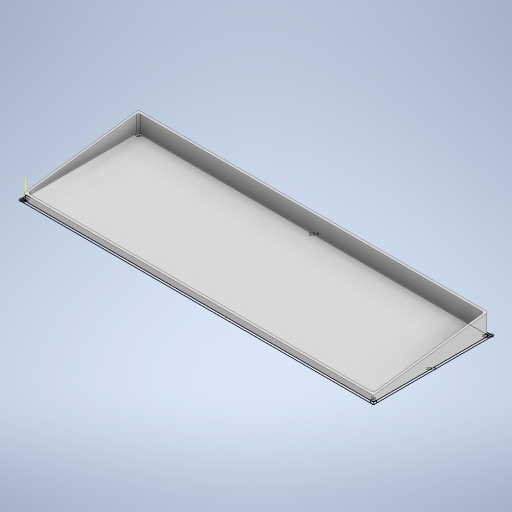
# Autodesk Inventor part: case_in_one
Saved by Autodesk Inventor 2024 (Build 280153000, 153)
## iProperties
Created: 2023-08-03
Part Number: case_in_one
Material: Generic
Document SubType Name: Modeling
Designer: Mika
Density: 1 g/cm^3
Appearance: Default
Author: Mika
Autodesk Inventor part; units mm, degrees
ref_plane "YZ Plane" through (0, 0, 0) normal (1, 0, 0) x (0, 1, 0)
ref_plane "XZ Plane" through (0, 0, 0) normal (0, 1, 0) x (-1, 0, 0)
ref_plane "XY Plane" through (0, 0, 0) normal (0, 0, 1) x (1, 0, 0)
sketch "Sketch1" plane through (0, 0, 0) normal (0, 1, 0) x (-1, 0, 0)
  line L0 (0, 0) -> (-2, 0)
  line L1 (-2, 0) -> (-2, -2)
  line L2 (-2, -2) -> (0, -2)
  line L3 (0, -2) -> (0, 0)
  line L4 (-2, -2) -> (-310.9, -2)
  line L5 (-310.9, -2) -> (-310.9, -103.5)
  line L6 (-308.9, -103.5) -> (-2, -103.5)
  line L7 (-2, -103.5) -> (-2, -2)
  line L8 (-310.9, -103.5) -> (-312.9, -103.5)
  line L9 (-312.9, -103.5) -> (-312.9, -105.5)
  line L10 (-312.9, -105.5) -> (-310.9, -105.5)
  line L11 (-310.9, -105.5) -> (-310.9, -103.5)
  line L12 (-312.9, -105.5) -> (0, -105.5)
  line L13 (0, -105.5) -> (0, 0)
  line L14 (0, 0) -> (-312.9, 0)
  line L15 (-312.9, 0) -> (-312.9, -105.5)
  line L16 (-2, -2) -> (-4, -2)
  line L17 (-4, -2) -> (-4, -4)
  line L18 (-4, -4) -> (-2, -4)
  line L19 (-2, -4) -> (-2, -2)
  line L20 (-2, -103.5) -> (-4, -103.5)
  line L21 (-4, -103.5) -> (-4, -101.5)
  line L22 (-4, -101.5) -> (-2, -101.5)
  line L23 (-2, -101.5) -> (-2, -103.5)
  line L24 (-310.9, -103.5) -> (-308.9, -103.5)
  line L25 (-308.9, -103.5) -> (-308.9, -101.5)
  line L26 (-308.9, -101.5) -> (-310.9, -101.5)
  line L27 (-310.9, -101.5) -> (-310.9, -103.5)
  line L28 (-310.9, -2) -> (-308.9, -2)
  line L29 (-308.9, -2) -> (-308.9, -4)
  line L30 (-308.9, -4) -> (-310.9, -4)
  line L31 (-310.9, -4) -> (-310.9, -2)
  circle A0 centre (-4, -101.5) radius 2
  circle A1 centre (-4, -4) radius 2
  circle A2 centre (-308.9, -4) radius 2
  circle A3 centre (-308.9, -101.5) radius 2
  circle A4 centre (-310.9, -103.5) radius 2
  circle A5 centre (-2, -103.5) radius 2
  circle A6 centre (-2, -2) radius 2
  circle A7 centre (-310.9, -2) radius 2
  point P0 (-2, -105.5)
  point P1 (0, -103.5)
  point P2 (-310.9, 0)
  point P3 (-312.9, -2)
  dimension "d0" = 2
  dimension "d1" = 2
  dimension "d2" = 308.9
  dimension "d3" = 101.5
  dimension "d4" = 2
  dimension "d5" = 2
  dimension "d6" = 2
  dimension "d7" = 2
  dimension "d8" = 2
  dimension "d9" = 2
  dimension "d10" = 2
  dimension "d11" = 2
  dimension "d12" = 2
  dimension "d13" = 2
  constraints: 64 end point, 16 parallel, 8 coincident, 8 horizontal, 8 perpendicular, 2 centre point, 2 tangent, 18 other
  measures "d0" distance of L2.end L1.end
  measures "d1" distance of L1.end L0.end
  measures "d2" distance of L6.end L5.end
  measures "d3" distance of L5.end L4.end
  measures "d4" distance of L10.end L9.end
  measures "d5" distance of L9.end L8.end
  measures "d6" distance of L18.end L17.end
  measures "d7" distance of L17.end L16.end
  measures "d8" distance of L21.end L22.end
  measures "d9" distance of L20.end L21.end
  measures "d10" distance of L26.end L25.end
  measures "d11" distance of L6.start L25.end
  measures "d12" distance of L29.end L30.end
  measures "d13" distance of L28.end L29.end
extrude "Extrusion1" add sketch "Sketch1" along normal blind 3 contours A1 L7 A0 L6 A3 L5 A2 L4 | A6 L18 L17 | L17 L18 A1 | A1 A6 | A2 L30 L29 | A7 A2 | L29 L30 A7 | A5 L21 L22 | L22 L21 A0 | A0 A5 | A3 L25 L26 | A4 A3 | L26 L25 A4
sketch "Sketch2" plane through (0, 3, 0) normal (0, 1, 0) x (1, 0, 0)
  arc A0 (2, 4) -> (4, 2) centre (4, 4) ccw projected
  line L0 (2, 2) -> (4, 2)
  line L1 (4, 2) -> (4, 4)
  line L2 (4, 4) -> (2, 4)
  line L3 (2, 4) -> (2, 2)
  arc A1 (310.9, 101.5) -> (308.9, 103.5) centre (308.9, 101.5) ccw projected
  line L4 (308.9, 101.5) -> (310.9, 101.5)
  line L5 (310.9, 101.5) -> (310.9, 103.5)
  line L6 (310.9, 103.5) -> (308.9, 103.5)
  line L7 (308.9, 103.5) -> (308.9, 101.5)
  line L8 (308.9, 101.5) -> (4, 101.5)
  line L9 (4, 101.5) -> (4, 4)
  line L10 (4, 4) -> (308.9, 4)
  line L11 (308.9, 4) -> (308.9, 101.5)
  line L12 (4, 101.5) -> (6, 101.5)
  line L13 (6, 101.5) -> (6, 99.5)
  line L14 (6, 99.5) -> (4, 99.5)
  line L15 (4, 99.5) -> (4, 101.5)
  line L16 (4, 4) -> (6, 4)
  line L17 (6, 4) -> (6, 6)
  line L18 (6, 6) -> (4, 6)
  line L19 (4, 6) -> (4, 4)
  line L20 (308.9, 4) -> (306.9, 4)
  line L21 (306.9, 4) -> (306.9, 6)
  line L22 (306.9, 6) -> (308.9, 6)
  line L23 (308.9, 6) -> (308.9, 4)
  line L24 (308.9, 101.5) -> (306.9, 101.5)
  line L25 (306.9, 101.5) -> (306.9, 99.5)
  line L26 (306.9, 99.5) -> (308.9, 99.5)
  line L27 (308.9, 99.5) -> (308.9, 101.5)
  circle A2 centre (306.9, 99.5) radius 2
  circle A3 centre (306.9, 6) radius 2
  circle A4 centre (6, 6) radius 2
  circle A5 centre (6, 99.5) radius 2
  line L28 (2, 2) -> (310.9, 2)
  line L29 (310.9, 2) -> (310.9, 103.5)
  line L30 (310.9, 103.5) -> (2, 103.5)
  line L31 (2, 103.5) -> (2, 2)
  point P0 (0, 0)
  dimension "d18" = 2
  dimension "d19" = 2
  dimension "d20" = 2
  dimension "d21" = 2
  dimension "d22" = 2
  dimension "d23" = 2
  dimension "d24" = 2
  dimension "d25" = 2
  constraints: 64 end point, 16 parallel, 8 horizontal, 8 perpendicular, 4 coincident, 12 other
  measures "d18" distance of L13.end L14.end
  measures "d19" distance of L12.end L13.end
  measures "d20" distance of L18.end L17.end
  measures "d21" distance of L17.end L16.end
  measures "d22" distance of L21.end L22.end
  measures "d23" distance of L20.end L21.end
  measures "d24" distance of L26.end L25.end
  measures "d25" distance of L25.end L24.end
extrude "Extrusion3" add sketch "Sketch2" along normal blind 15 contours L2 L1 A0 | L31 L30 L7 L8 L9 L2 | L1 L10 L11 L4 L29 L28 | L9 A4 L10 | A1 L4 L7 | L9 L8 A5 | A3 L11 L10 | L11 A2 L8
sketch "Sketch6" plane through (4, 0, -2) normal (0, 0, 1) x (1, 0, 0)
  line L0 (0, 0) -> (0, 5)
  line L1 (0, 0) -> (0, 18) projected
  line L2 (0, 5) -> (4.2844, 5)
  point P0 (-4, 0)
  dimension "d30" = 5
  constraints: 4 end point, 1 horizontal, 1 point on line
  measures "d30" distance of L0.start L0.end
ref_plane "Work Plane3" through (4, 5, -2) normal (0, 0.9918975, 0.1270411) x (1, 0, 0)
sketch "Sketch7" plane through (4, 5, -2) normal (0, 0.9918975, 0.1270411) x (1, 0, 0)
  line L0 (-11.9738, -4.1183) -> (314.319, -4.1183)
  line L1 (314.319, -4.1183) -> (314.319, 105.2243)
  line L2 (314.319, 105.2243) -> (-11.9738, 105.2243)
  line L3 (-11.9738, 105.2243) -> (-11.9738, -4.1183)
  point P0 (-4, -2.619)
  constraints: 8 end point, 2 parallel, 1 horizontal, 1 perpendicular
extrude "Extrusion4" cut sketch "Sketch7" along normal blind 15
body "Solid1"
